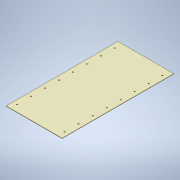
# Autodesk Inventor part: top_bottom_layer_3mm
Saved by Autodesk Inventor 2021 (Build 250183000, 183)
## iProperties
Created: 2021-01-27
Part Number: top_bottom_layer_3mm
Material: Acrylic
Document SubType Name: Modeling
Designer: abij996
Density: 1.188 g/cm^3
Appearance: Smooth - Ash
Author: abij996
Autodesk Inventor part; units mm, degrees
ref_plane "YZ Plane" through (0, 0, 0) normal (1, 0, 0) x (0, 1, 0)
ref_plane "XZ Plane" through (0, 0, 0) normal (0, 1, 0) x (-1, 0, 0)
ref_plane "XY Plane" through (0, 0, 0) normal (0, 0, 1) x (1, 0, 0)
sketch "Sketch2" plane through (0, 0, 0) normal (0, 1, 0) x (-1, 0, 0)
  line L0 (238.7833, 365.019) -> (-161.2167, 365.019)
  line L1 (-161.2167, 365.019) -> (-161.2167, -434.981)
  line L2 (-161.2167, -434.981) -> (238.7833, -434.981)
  line L3 (238.7833, -434.981) -> (238.7833, 365.019)
  circle A0 centre (208.7833, 217.5648) radius 4
  circle A1 centre (208.7833, 317.5648) radius 4
  circle A2 centre (209.7833, -382.4352) radius 4
  circle A3 centre (209.7833, -283.981) radius 4
  circle A4 centre (209.7833, -183.981) radius 4
  circle A5 centre (209.7833, -83.981) radius 4
  circle A6 centre (209.7833, 16.019) radius 4
  circle A7 centre (209.7833, 116.019) radius 4
  line L4 (38.7833, -434.981) -> (38.7833, 365.019) construction
  circle A8 centre (-131.2167, 217.5648) radius 4
  circle A9 centre (-132.2167, 16.019) radius 4
  circle A10 centre (-132.2167, 116.019) radius 4
  circle A11 centre (-132.2167, -382.4352) radius 4
  circle A12 centre (-132.2167, -283.981) radius 4
  circle A13 centre (-132.2167, -183.981) radius 4
  circle A14 centre (-132.2167, -83.981) radius 4
  circle A15 centre (-131.2167, 317.5648) radius 4
  point P0 (0, 0)
  dimension "d46" = 800
  dimension "d47" = 400
  dimension "d74" = 8
  dimension "d75" = 8
  dimension "d77" = 8
  dimension "d78" = 8
  dimension "d79" = 8
  dimension "d80" = 8
  dimension "d81" = 8
  constraints: 16 centre point, 10 end point, 8 symmetric about line, 2 midpoint, 2 parallel, 1 horizontal, 1 perpendicular, 8 other
  measures "d46" distance of L2.end L0.start
  measures "d47" distance of L0.start L0.end
  measures "d74" diameter of A0
  measures "d75" diameter of A1
  measures "d77" diameter of A3
  measures "d78" diameter of A4
  measures "d79" diameter of A5
  measures "d80" diameter of A6
  measures "d81" diameter of A7
extrude "Extrusion7" add sketch "Sketch2" along normal blind 3
body "Solid7"
